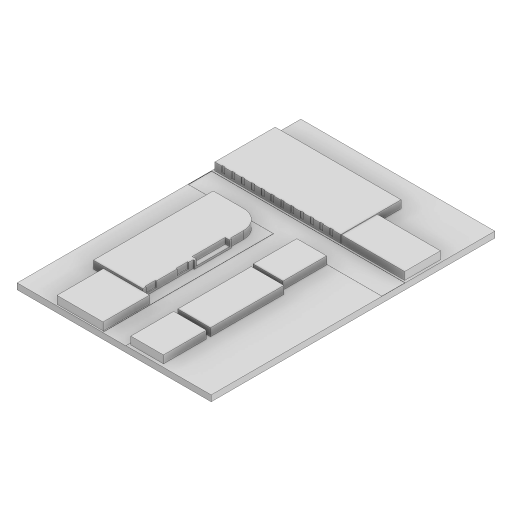
# Autodesk Inventor part: T_intersection
Saved by Autodesk Inventor 2023 (Build 270158000, 158)
## iProperties
Created: 2022-07-11
Part Number: T_intersection
Material: Generic
Document SubType Name: Modeling
Designer: Derm
Density: 1 g/cm^3
Appearance: Default
Author: Derm
Autodesk Inventor part; units mm, degrees
ref_plane "YZ Plane" through (0, 0, 0) normal (1, 0, 0) x (0, 1, 0)
ref_plane "XZ Plane" through (0, 0, 0) normal (0, 1, 0) x (-1, 0, 0)
ref_plane "XY Plane" through (0, 0, 0) normal (0, 0, 1) x (1, 0, 0)
sketch "Sketch1" plane through (0, 0, 0) normal (0, 1, 0) x (-1, 0, 0)
  line L0 (-6000, 15000) -> (6000, 15000)
  line L1 (6000, 15000) -> (6000, -15000)
  line L2 (6000, -15000) -> (-6000, -15000)
  line L3 (-6000, -15000) -> (-6000, 15000)
  line L4 (-6000, 15000) -> (6000, -15000) construction
  line L5 (6000, 15000) -> (-6000, -15000) construction
  line L6 (-50000, -27000) -> (50000, -27000)
  line L7 (50000, -27000) -> (50000, -15000)
  line L8 (50000, -15000) -> (-50000, -15000)
  line L9 (-50000, -15000) -> (-50000, -27000)
  line L10 (-50000, -27000) -> (50000, -15000) construction
  line L11 (50000, -27000) -> (-50000, -15000) construction
  line L12 (6000, 15000) -> (-6000, 15000)
  line L13 (-6000, 15000) -> (-6000, 73309.9915)
  line L14 (-6000, 73309.9915) -> (6000, 73309.9915)
  line L15 (6000, 73309.9915) -> (6000, 15000)
  point P0 (0, 0)
  point P1 (0, -21000)
  dimension "d0" = 30000
  dimension "d1" = 12000
  dimension "d2" = 12000
  dimension "d3" = 100000
  constraints: 32 end point, 6 parallel, 4 midpoint, 3 horizontal, 3 perpendicular, 1 collinear
  measures "d0" distance of L0.end L1.end
  measures "d1" distance of L1.end L2.end
  measures "d2" distance of L6.end L7.end
  measures "d3" distance of L6.start L6.end
extrude "Extrusion1" add sketch "Sketch1" against normal blind 25.4
sketch "Sketch2" plane through (0, 0, 0) normal (0, 1, 0) x (-1, 0, 0)
  line L0 (-6000, 73309.9915) -> (-6000, -15000) projected
  line L1 (-6000, -15000) -> (-50000, -15000) projected
  line L2 (-50000, -15000) -> (-50000, -27000) projected
  line L3 (-50000, -27000) -> (50000, -27000) projected
  line L4 (50000, -27000) -> (50000, -15000) projected
  line L5 (50000, -15000) -> (6000, -15000) projected
  line L6 (6000, -15000) -> (6000, 73309.9915) projected
  line L7 (6000, 73309.9915) -> (-6000, 73309.9915) projected
  line L8 (-50098.5986, -73309.9915) -> (50189.0701, -73309.9915)
  line L9 (50189.0701, -73309.9915) -> (50189.0701, 73309.9915)
  line L10 (50189.0701, 73309.9915) -> (-50098.5986, 73309.9915)
  line L11 (-50098.5986, 73309.9915) -> (-50098.5986, -73309.9915)
  point P0 (0, 0)
  constraints: 8 end point, 2 parallel, 1 collinear, 1 horizontal
extrude "Extrusion2" add sketch "Sketch2" along normal blind 101.6 contours L0 L1 L2 L3 L4 L5 L6 L10 L9 L8 L11
sketch "Sketch3" plane through (0, 101.6, 0) normal (0, 1, 0) x (1, 0, 0)
  line L0 (-6000, -73309.9915) -> (-6000, 15000) projected
  line L1 (-6000, 15000) -> (-50000, 15000) projected
  line L2 (-50000, 15000) -> (-50000, 27000) projected
  line L3 (-50000, 27000) -> (50000, 27000) projected
  line L4 (50000, 27000) -> (50000, 15000) projected
  line L5 (50000, 15000) -> (6000, 15000) projected
  line L6 (6000, 15000) -> (6000, -73309.9915) projected
  line L7 (6000, -73309.9915) -> (50098.5986, -73309.9915) projected
  line L8 (50098.5986, -73309.9915) -> (50098.5986, 73309.9915) projected
  line L9 (50098.5986, 73309.9915) -> (-50189.0701, 73309.9915) projected
  line L10 (-50189.0701, 73309.9915) -> (-50189.0701, -73309.9915) projected
  line L11 (-50189.0701, -73309.9915) -> (-6000, -73309.9915) projected
  line L12 (6306.6835, 14762.6658) -> (21728.0263, 14762.6658)
  line L13 (21728.0263, 14762.6658) -> (21728.0263, -7819.4322)
  line L14 (21728.0263, -7819.4322) -> (6306.6835, -7819.4322)
  line L15 (6306.6835, -7819.4322) -> (6306.6835, 14762.6658)
  line L16 (7008.1027, -9506.0891) -> (23874.6817, -9506.0891)
  line L17 (23874.6817, -9506.0891) -> (23874.6817, -47455.8921)
  line L18 (23874.6817, -47455.8921) -> (7008.1027, -47455.8921)
  line L19 (7008.1027, -47455.8921) -> (7008.1027, -9506.0891)
  line L20 (7008.1027, -49602.5476) -> (23874.6817, -49602.5476)
  line L21 (23874.6817, -49602.5476) -> (23874.6817, -71759.0992)
  line L22 (23874.6817, -71759.0992) -> (7008.1027, -71759.0992)
  line L23 (7008.1027, -71759.0992) -> (7008.1027, -49602.5476)
  line L24 (-21096.9853, 14530.3509) -> (-36663.68, 14530.3509)
  line L25 (-36663.68, 14530.3509) -> (-36663.68, -47455.8921)
  line L26 (-36663.68, -47455.8921) -> (-11096.9853, -47455.8921)
  line L27 (-11096.9853, -47455.8921) -> (-11096.9853, 4530.3509)
  arc A0 (-11096.9853, 4530.3509) -> (-21096.9853, 14530.3509) centre (-21096.9853, 4530.3509) ccw
  line L28 (-6488.4065, -48575.3194) -> (-30308.5337, -48575.3194)
  line L29 (-30308.5337, -48575.3194) -> (-30308.5337, -72602.7202)
  line L30 (-30308.5337, -72602.7202) -> (-6488.4065, -72602.7202)
  line L31 (-6488.4065, -72602.7202) -> (-6488.4065, -48575.3194)
  line L32 (-11096.9853, -21462.7706) -> (-10448.8665, -21462.7706)
  line L33 (-10448.8665, -21462.7706) -> (-10448.8665, -2230.0491)
  line L34 (-10448.8665, -2230.0491) -> (-11096.9853, -2230.0491)
  line L35 (-11096.9853, -2230.0491) -> (-11096.9853, -21462.7706)
  line L36 (-49233.7439, 27939.6609) -> (15844.5264, 27939.6609)
  line L37 (15844.5264, 27939.6609) -> (15844.5264, 59114.4404)
  line L38 (15844.5264, 59114.4404) -> (-49233.7439, 59114.4404)
  line L39 (-49233.7439, 59114.4404) -> (-49233.7439, 27939.6609)
  line L40 (16150.2544, 27939.6609) -> (48849.1686, 27939.6609)
  line L41 (48849.1686, 27939.6609) -> (48849.1686, 46468.0676)
  line L42 (48849.1686, 46468.0676) -> (16150.2544, 46468.0676)
  line L43 (16150.2544, 46468.0676) -> (16150.2544, 27939.6609)
  point P0 (0, 0)
  point P1 (-11096.9853, -2230.0491)
  dimension "d8" = 10000
  constraints: 64 end point, 16 parallel, 8 horizontal, 8 perpendicular, 3 point on line, 2 point on circle, 2 tangent, 1 centre point, 1 midpoint
  measures "d8" radius of A0
extrude "Extrusion3" add sketch "Sketch3" along normal blind 4000 contours L12 L13 L14 L15 | L16 L17 L18 L19 | L20 L21 L22 L23 | A0 L27 L26 L25 L24 | L34 L33 L32 L27 | L31 L30 L29 L28 | L39 L38 L37 L36 | L43 L42 L41 L40
sketch "Sketch4" plane through (0, 4101.6, 0) normal (0, 1, 0) x (1, 0, 0)
  line L0 (15844.5264, 27939.6609) -> (15844.5264, 59114.4404)
  line L1 (15844.5264, 59114.4404) -> (-49233.7439, 59114.4404)
  line L2 (-49233.7439, 59114.4404) -> (-49233.7439, 27939.6609)
  line L3 (-49233.7439, 27939.6609) -> (15844.5264, 27939.6609)
  line L4 (48849.1686, 27939.6609) -> (48849.1686, 46468.0676)
  line L5 (48849.1686, 46468.0676) -> (16150.2544, 46468.0676)
  line L6 (16150.2544, 46468.0676) -> (16150.2544, 27939.6609)
  line L7 (16150.2544, 27939.6609) -> (48849.1686, 27939.6609)
  line L8 (6306.6835, -7819.4322) -> (21728.0263, -7819.4322)
  line L9 (21728.0263, -7819.4322) -> (21728.0263, 14762.6658)
  line L10 (21728.0263, 14762.6658) -> (6306.6835, 14762.6658)
  line L11 (6306.6835, 14762.6658) -> (6306.6835, -7819.4322)
  line L12 (-11096.9853, -47455.8921) -> (-11096.9853, -21462.7706)
  line L13 (-11096.9853, -21462.7706) -> (-10448.8665, -21462.7706)
  line L14 (-10448.8665, -21462.7706) -> (-10448.8665, -2230.0491)
  line L15 (-10448.8665, -2230.0491) -> (-11096.9853, -2230.0491)
  line L16 (-11096.9853, -2230.0491) -> (-11096.9853, 4530.3509)
  arc A0 (-11096.9853, 4530.3509) -> (-21096.9853, 14530.3509) centre (-21096.9853, 4530.3509) ccw
  line L17 (-21096.9853, 14530.3509) -> (-36663.68, 14530.3509)
  line L18 (-36663.68, 14530.3509) -> (-36663.68, -47455.8921)
  line L19 (-36663.68, -47455.8921) -> (-11096.9853, -47455.8921)
  line L20 (7008.1027, -47455.8921) -> (23874.6817, -47455.8921)
  line L21 (23874.6817, -47455.8921) -> (23874.6817, -9506.0891)
  line L22 (23874.6817, -9506.0891) -> (7008.1027, -9506.0891)
  line L23 (7008.1027, -9506.0891) -> (7008.1027, -47455.8921)
  line L24 (-30308.5337, -48575.3194) -> (-30308.5337, -72602.7202)
  line L25 (-30308.5337, -72602.7202) -> (-6488.4065, -72602.7202)
  line L26 (-6488.4065, -72602.7202) -> (-6488.4065, -48575.3194)
  line L27 (-6488.4065, -48575.3194) -> (-30308.5337, -48575.3194)
  line L28 (7008.1027, -71759.0992) -> (23874.6817, -71759.0992)
  line L29 (23874.6817, -71759.0992) -> (23874.6817, -49602.5476)
  line L30 (23874.6817, -49602.5476) -> (7008.1027, -49602.5476)
  line L31 (7008.1027, -49602.5476) -> (7008.1027, -71759.0992)
  line L32 (10161.3604, 27939.6609) -> (11714.5969, 27939.6609)
  line L33 (11714.5969, 27939.6609) -> (11714.5969, 28261.1616)
  line L34 (11714.5969, 28261.1616) -> (10161.3604, 28261.1616)
  line L35 (10161.3604, 28261.1616) -> (10161.3604, 27939.6609)
  line L36 (6634.5969, 28261.1616) -> (5081.3604, 28261.1616)
  line L37 (5081.3604, 28261.1616) -> (5081.3604, 27939.6609)
  line L38 (5081.3604, 27939.6609) -> (6634.5969, 27939.6609)
  line L39 (6634.5969, 27939.6609) -> (6634.5969, 28261.1616)
  line L40 (1554.5969, 28261.1616) -> (1.3604, 28261.1616)
  line L41 (1.3604, 28261.1616) -> (1.3604, 27939.6609)
  line L42 (1.3604, 27939.6609) -> (1554.5969, 27939.6609)
  line L43 (1554.5969, 27939.6609) -> (1554.5969, 28261.1616)
  line L44 (-3525.4031, 28261.1616) -> (-5078.6396, 28261.1616)
  line L45 (-5078.6396, 28261.1616) -> (-5078.6396, 27939.6609)
  line L46 (-5078.6396, 27939.6609) -> (-3525.4031, 27939.6609)
  line L47 (-3525.4031, 27939.6609) -> (-3525.4031, 28261.1616)
  line L48 (-8605.4031, 28261.1616) -> (-10158.6396, 28261.1616)
  line L49 (-10158.6396, 28261.1616) -> (-10158.6396, 27939.6609)
  line L50 (-10158.6396, 27939.6609) -> (-8605.4031, 27939.6609)
  line L51 (-8605.4031, 27939.6609) -> (-8605.4031, 28261.1616)
  line L52 (-13685.4031, 28261.1616) -> (-15238.6396, 28261.1616)
  line L53 (-15238.6396, 28261.1616) -> (-15238.6396, 27939.6609)
  line L54 (-15238.6396, 27939.6609) -> (-13685.4031, 27939.6609)
  line L55 (-13685.4031, 27939.6609) -> (-13685.4031, 28261.1616)
  line L56 (-18765.4031, 28261.1616) -> (-20318.6396, 28261.1616)
  line L57 (-20318.6396, 28261.1616) -> (-20318.6396, 27939.6609)
  line L58 (-20318.6396, 27939.6609) -> (-18765.4031, 27939.6609)
  line L59 (-18765.4031, 27939.6609) -> (-18765.4031, 28261.1616)
  line L60 (-23845.4031, 28261.1616) -> (-25398.6396, 28261.1616)
  line L61 (-25398.6396, 28261.1616) -> (-25398.6396, 27939.6609)
  line L62 (-25398.6396, 27939.6609) -> (-23845.4031, 27939.6609)
  line L63 (-23845.4031, 27939.6609) -> (-23845.4031, 28261.1616)
  line L64 (-28925.4031, 28261.1616) -> (-30478.6396, 28261.1616)
  line L65 (-30478.6396, 28261.1616) -> (-30478.6396, 27939.6609)
  line L66 (-30478.6396, 27939.6609) -> (-28925.4031, 27939.6609)
  line L67 (-28925.4031, 27939.6609) -> (-28925.4031, 28261.1616)
  line L68 (-34005.4031, 28261.1616) -> (-35558.6396, 28261.1616)
  line L69 (-35558.6396, 28261.1616) -> (-35558.6396, 27939.6609)
  line L70 (-35558.6396, 27939.6609) -> (-34005.4031, 27939.6609)
  line L71 (-34005.4031, 27939.6609) -> (-34005.4031, 28261.1616)
  line L72 (-39085.4031, 28261.1616) -> (-40638.6396, 28261.1616)
  line L73 (-40638.6396, 28261.1616) -> (-40638.6396, 27939.6609)
  line L74 (-40638.6396, 27939.6609) -> (-39085.4031, 27939.6609)
  line L75 (-39085.4031, 27939.6609) -> (-39085.4031, 28261.1616)
  line L76 (-44165.4031, 28261.1616) -> (-45718.6396, 28261.1616)
  line L77 (-45718.6396, 28261.1616) -> (-45718.6396, 27939.6609)
  line L78 (-45718.6396, 27939.6609) -> (-44165.4031, 27939.6609)
  line L79 (-44165.4031, 27939.6609) -> (-44165.4031, 28261.1616)
  point P0 (0, 0)
extrude "Extrusion4" cut sketch "Sketch4" against normal blind 3000 contours L3 L35 L34 L33 | L3 L37 L36 L39 | L77 L76 L79 L3 | L3 L41 L40 L43 | L73 L72 L75 L3 | L3 L45 L44 L47 | L69 L68 L71 L3 | L3 L49 L48 L51 | L65 L64 L67 L3 | L3 L53 L52 L55 | L61 L60 L63 L3 | L3 L57 L56 L59
sketch "Sketch5" plane through (0, 4101.6, 0) normal (0, 1, 0) x (1, 0, 0)
  line L0 (-11096.9853, -47455.8921) -> (-11096.9853, -21462.7706) projected
  line L1 (-11096.9853, -21462.7706) -> (-10448.8665, -21462.7706) projected
  line L2 (-10448.8665, -21462.7706) -> (-10448.8665, -2230.0491) projected
  line L3 (-10448.8665, -2230.0491) -> (-11096.9853, -2230.0491) projected
  line L4 (-11096.9853, -2230.0491) -> (-11096.9853, 4530.3509) projected
  arc A0 (-11096.9853, 4530.3509) -> (-21096.9853, 14530.3509) centre (-21096.9853, 4530.3509) ccw projected
  line L5 (-21096.9853, 14530.3509) -> (-36663.68, 14530.3509) projected
  line L6 (-36663.68, 14530.3509) -> (-36663.68, -47455.8921) projected
  line L7 (-36663.68, -47455.8921) -> (-11096.9853, -47455.8921) projected
  line L8 (-12765.877, -3225.5553) -> (-10448.8665, -3225.5553)
  line L9 (-10448.8665, -3225.5553) -> (-10448.8665, -20314.1354)
  line L10 (-10448.8665, -20314.1354) -> (-12765.877, -20314.1354)
  line L11 (-12765.877, -20314.1354) -> (-12765.877, -3225.5553)
  line L12 (-11096.9853, -21462.7706) -> (-11096.9853, -47455.8921) projected
  line L13 (-11096.9853, -45801.5963) -> (-11607.3718, -45801.5963)
  line L14 (-11607.3718, -45801.5963) -> (-11607.3718, -40517.1763)
  line L15 (-11607.3718, -40517.1763) -> (-11096.9853, -40517.1763)
  line L16 (-11096.9853, -40517.1763) -> (-11096.9853, -45801.5963)
  line L17 (-11096.9853, -29742.4496) -> (-11607.3718, -29742.4496)
  line L18 (-11607.3718, -29742.4496) -> (-11607.3718, -23771.7412)
  line L19 (-11607.3718, -23771.7412) -> (-11096.9853, -23771.7412)
  line L20 (-11096.9853, -23771.7412) -> (-11096.9853, -29742.4496)
  point P0 (0, 0)
  constraints: 24 end point, 6 parallel, 4 point on line, 3 horizontal, 3 perpendicular
extrude "Extrusion5" cut sketch "Sketch5" against normal blind 3000 contours L13 L14 L15 L0 | L17 L18 L19 L0 | L10 L11 L8 L2
sketch "Sketch6" plane through (0, 0, 0) normal (0, -1, 0) x (1, 0, 0)
  line L0 (-6000, -15000) -> (-6000, 73309.9915) projected
  line L1 (-50189.0701, 73309.9915) -> (-6000, 73309.9915) projected
  line L2 (-50189.0701, -73309.9915) -> (-50189.0701, 73309.9915) projected
  line L3 (50098.5986, -73309.9915) -> (-50189.0701, -73309.9915) projected
  line L4 (50098.5986, 73309.9915) -> (50098.5986, -73309.9915) projected
  line L5 (6000, 73309.9915) -> (50098.5986, 73309.9915) projected
  line L6 (6000, 73309.9915) -> (6000, -15000) projected
  line L7 (6000, -15000) -> (50000, -15000) projected
  line L8 (50000, -15000) -> (50000, -27000) projected
  line L9 (50000, -27000) -> (-50000, -27000) projected
  line L10 (-50000, -27000) -> (-50000, -15000) projected
  line L11 (-50000, -15000) -> (-6000, -15000) projected
  line L12 (6000, -15000) -> (6000, 73309.9915) projected
  line L13 (6000, 73309.9915) -> (-6000, 73309.9915) projected
  line L14 (-6000, 73309.9915) -> (-6000, -15000) projected
  line L15 (-6000, -15000) -> (-50000, -15000) projected
  line L16 (-50000, -15000) -> (-50000, -27000) projected
  line L17 (-50000, -27000) -> (50000, -27000) projected
  line L18 (50000, -27000) -> (50000, -15000) projected
  line L19 (50000, -15000) -> (6000, -15000) projected
  point P0 (0, 0)
  point P1 (-6000, 73309.9915)
extrude "Extrusion6" add sketch "Sketch6" along normal blind 3000
body "Solid1"
